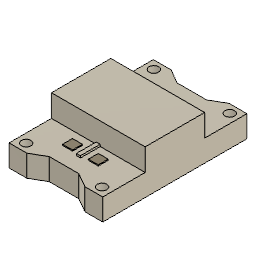
SPARK Rev (Autodesk Fusion 360 design; units mm, degrees)
part number: 2026-02-17-14-50-15-895
Autodesk Fusion 360 part; units mm, degrees
sketch "Sketch1" plane through (0, 0, 0) normal (0, 0, 1) x (1, 0, 0)
  line L0 (47.3, 0) -> (47.3, 72.8)
  line L1 (0, 72.8) -> (0, 0)
  circle A0 centre (4.51, 4.21) radius 2.41
  line L2 (0, 36.4) -> (47.3, 36.4) construction
  line L3 (0, 21.4) -> (47.3, 21.4)
  line L4 (23.65, 72.8) -> (23.65, -0.0931) construction
  line L5 (16.2, 4.1569) -> (31.1, 4.1569)
  line L6 (16.2, 4.1569) -> (9, 0)
  line L7 (31.1, 4.1569) -> (38.3, 0)
  circle A1 centre (42.79, 4.21) radius 2.41
  line L8 (0, 0) -> (9, 0)
  line L9 (38.3, 0) -> (47.3, 0)
  line L10 (0, 72.8) -> (47.3, 72.8) construction
  line L11 (22.65, 21.4) -> (24.65, 21.4)
  line L12 (24.65, 21.4) -> (24.65, 11.4)
  line L13 (24.65, 11.4) -> (22.65, 11.4)
  line L14 (22.65, 11.4) -> (22.65, 21.4)
  line L15 (19.65, 17.4) -> (14.65, 17.4)
  line L16 (14.65, 17.4) -> (14.65, 12.4)
  line L17 (14.65, 12.4) -> (19.65, 12.4)
  line L18 (19.65, 12.4) -> (19.65, 17.4)
  line L19 (32.65, 12.4) -> (27.65, 12.4)
  line L20 (27.65, 12.4) -> (27.65, 17.4)
  line L21 (32.65, 17.4) -> (32.65, 12.4)
  line L22 (27.65, 17.4) -> (32.65, 17.4)
  line L23 (16.2, 68.6431) -> (31.1, 68.6431)
  line L24 (14.65, 55.4) -> (14.65, 60.4)
  line L25 (38.3, 72.8) -> (47.3, 72.8)
  line L26 (24.65, 51.4) -> (24.65, 61.4)
  line L27 (27.65, 60.4) -> (27.65, 55.4)
  line L28 (22.65, 61.4) -> (22.65, 51.4)
  line L29 (16.2, 68.6431) -> (9, 72.8)
  line L30 (19.65, 60.4) -> (19.65, 55.4)
  line L31 (32.65, 60.4) -> (27.65, 60.4)
  line L32 (31.1, 68.6431) -> (38.3, 72.8)
  line L33 (19.65, 55.4) -> (14.65, 55.4)
  line L34 (14.65, 60.4) -> (19.65, 60.4)
  line L35 (24.65, 61.4) -> (22.65, 61.4)
  circle A2 centre (42.79, 68.59) radius 2.41
  line L36 (32.65, 55.4) -> (32.65, 60.4)
  line L37 (0, 72.8) -> (9, 72.8)
  line L38 (23.65, 0) -> (23.65, 72.8931) construction
  line L39 (27.65, 55.4) -> (32.65, 55.4)
  circle A3 centre (4.51, 68.59) radius 2.41
  line L40 (0, 51.4) -> (47.3, 51.4)
  point P0 (23.65, 4.1569)
  point P1 (23.65, 21.4)
  point P2 (0, 72.8)
  point P3 (23.65, 68.6431)
  dimension "d1" = 47.3
  dimension "d2" = 72.8
  dimension "d3" = 4.82
  dimension "d4" = 4.51
  dimension "d5" = 4.21
  dimension "d6" = 15
  dimension "d7" = 16.2
  dimension "d8" = 4.25
  dimension "d9" = 30
  dimension "d10" = 9
  dimension "d11" = 2
  dimension "d12" = 10
  dimension "d13" = 5
  dimension "d14" = 5
  dimension "d15" = 4
  dimension "d16" = 4
  constraint horizontal L8
  constraint vertical L0
  constraint vertical L1
  constraint coincident L1.end L8.start
  constraint midpoint L1 L2.start
  constraint midpoint L0 L2.end
  constraint coincident L1 L3.start
  constraint coincident L0 L3.end
  constraint perpendicular L0 L3
  constraint midpoint L5 P0
  constraint coincident L4 P0
  constraint perpendicular L4 L5
  constraint symmetric A0 L4 A1
  constraint symmetric L4 L5.start L5.end
  constraint symmetric L4 L6.end L7.end
  constraint collinear L8 L9
  constraint horizontal P2 L4.start
  constraint midpoint L4.start L10
  constraint horizontal L11
  constraint vertical L12
  constraint horizontal L13
  constraint vertical L14
  constraint coincident L3 L11.start
  constraint midpoint L11 P1
  constraint coincident L4 P1
  constraint horizontal L15
  constraint vertical L16
  constraint horizontal L17
  constraint vertical L18
  constraint symmetric L4 L15.start L20.end
  constraint symmetric L4 L15.end L21.start
  constraint symmetric L4 L16.end L19.start
  constraint symmetric L4 L17.end L19.end
  constraint symmetric L1.end L2 P2
  constraint symmetric L0.start L2 L0.end
  constraint symmetric A0 L2 A3
  constraint symmetric L2 L3.start L40.start
  constraint symmetric L2 L3.end L40.end
  constraint symmetric L2 L4.start L38.start
  constraint symmetric L2 L4.end L38.end
  constraint symmetric L2 L5.start L23.start
  constraint symmetric L2 L5.end L23.end
  constraint symmetric L2 P0 P3
  constraint symmetric L2 L6.end L29.end
  constraint symmetric L2 L7.end L25.start
  constraint symmetric L2 A1 A2
  constraint symmetric L2 L11.start L28.end
  constraint symmetric L2 L11.end L26.start
  constraint symmetric L2 L12.end L26.end
  constraint symmetric L2 L13.end L28.start
  constraint symmetric L2 L15.start L30.end
  constraint symmetric L2 L15.end L24.start
  constraint symmetric L2 L16.end L24.end
  constraint symmetric L2 L17.end L30.start
  constraint symmetric L2 L19.start L31.start
  constraint symmetric L2 L19.end L27.start
  constraint symmetric L2 L20.end L27.end
  constraint symmetric L2 L21.start L36.start
  measures "d1" distance of L1.end L0.start
  measures "d2" distance of L1.end P2
  measures "d3" diameter of A0
  measures "d4" distance of L1 A0.centre
  measures "d5" vertical distance of L1.end A0.centre
  measures "d6" distance of L2 L3
  measures "d7" horizontal distance of L1.end L5.start
  measures "d8" distance of L4.end P0
  measures "d9" angle of L6 L8
  measures "d10" distance of L1.end L6.end
  measures "d11" distance of L11.start L11.end
  measures "d12" distance of L13 P1
  measures "d13" distance of L15.start L15.end
  measures "d14" distance of L15.start L17.end
  measures "d15" horizontal distance of P1 L15.start
  measures "d16" vertical distance of P1 L15.start
extrude "Extrude1" add sketch "Sketch1" along normal blind 22.2 contours L0 L1 L3 L11 L40
extrude "Extrude2" add sketch "Sketch1" along normal blind 12 contours L3 L11 L12 L13 L14 | L26 L28 L35 L40
extrude "Extrude3" add sketch "Sketch1" along normal blind 11 contours L0 L1 L3 L5 L6 L7 L8 L9 L12 L13 L14 | L0 L1 L23 L25 L26 L28 L29 L32 L35 L37 L40
extrude "Extrude4" add sketch "Sketch1" along normal blind 11.5 contours L15 L16 L17 L18 | L19 L20 L21 L22 | L24 L30 L33 L34 | L27 L31 L36 L39
equation "d4 = ( 4.82 / 2 ) * 1 mm + 2.1 mm"
equation "d5 = ( 4.82 / 2 ) * 1 mm + 1.8 mm"
